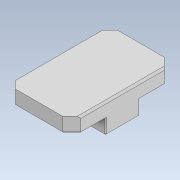
# Autodesk Inventor part: body_5
Saved by Autodesk Inventor 2020 (Build 240168000, 168)
## iProperties
Created: 2020-12-16
Part Number: body_5
Material: Generic
Document SubType Name: Modeling
Designer: DELL
Density: 1 g/cm^3
Appearance: Default
Mass: 2697.24 g
Surface Area: 1762.92 cm^2
Volume: 2697.24 cm^3
Author: DELL
Autodesk Inventor part; units mm, degrees
ref_plane "YZ Plane" through (0, 0, 0) normal (1, 0, 0) x (0, 1, 0)
ref_plane "XZ Plane" through (0, 0, 0) normal (0, 1, 0) x (-1, 0, 0)
ref_plane "XY Plane" through (0, 0, 0) normal (0, 0, 1) x (1, 0, 0)
sketch "Sketch1" plane through (0, 0, 0) normal (0, 1, 0) x (-1, 0, 0)
  line L0 (-90, -140) -> (90, -140)
  line L1 (90, -140) -> (90, 140)
  line L2 (90, 140) -> (-90, 140)
  line L3 (-90, 140) -> (-90, -140)
  line L4 (-90, -140) -> (90, 140) construction
  line L5 (90, -140) -> (-90, 140) construction
  point P0 (0, 0)
  dimension "d0" = 280
  dimension "d1" = 180
  constraints: 12 end point, 2 midpoint, 2 parallel, 1 horizontal, 1 perpendicular
  measures "d0" distance of L0.end L1.end
  measures "d1" distance between parallel lines of L3 L1
extrude "Extrusion1" add sketch "Sketch1" along normal blind 80
sketch "Sketch2" plane through (0, 0, 0) normal (0, -1, 0) x (1, 0, 0)
  arc A0 (-47.5, 47.5) -> (2.5, 97.5) centre (-47.5, 97.5) ccw
  line L0 (0, 150) -> (0, -153.5615) construction
  line L1 (-95.9498, 0) -> (75.0535, 0) construction
  line L2 (2.5, 97.5) -> (2.5, 140)
  line L3 (-90, 47.5) -> (-47.5, 47.5)
  line L4 (-90, -140) -> (-90, 140) projected
  line L5 (-90, 47.5) -> (-90, 140)
  line L6 (-90, 140) -> (90, 140) projected
  line L7 (2.5, 140) -> (-90, 140)
  arc A1 (-2.5, 97.5) -> (47.5, 47.5) centre (47.5, 97.5) ccw
  line L8 (-2.5, 97.5) -> (-2.5, 140)
  line L9 (90, 47.5) -> (47.5, 47.5)
  line L10 (90, -140) -> (90, 140)
  line L11 (90, 140) -> (-90, 140)
  arc A2 (2.5, -97.5) -> (-47.5, -47.5) centre (-47.5, -97.5) ccw
  line L12 (2.5, -97.5) -> (2.5, -140)
  line L13 (-90, -47.5) -> (-47.5, -47.5)
  line L14 (-90, 140) -> (-90, -140)
  line L15 (-90, -140) -> (90, -140)
  line L16 (90, 140) -> (90, -140)
  line L17 (90, -47.5) -> (47.5, -47.5)
  arc A3 (47.5, -47.5) -> (-2.5, -97.5) centre (47.5, -97.5) ccw
  line L18 (-2.5, -97.5) -> (-2.5, -140)
  circle A4 centre (-47.5, 97.5) radius 34.5
  circle A5 centre (-47.5, 97.5) radius 42 construction
  line L19 (-89.5, 97.5) -> (-5.5, 97.5) construction
  line L20 (-47.5, 139.5) -> (-47.5, 55.5) construction
  line L21 (-77.1985, 127.1985) -> (-17.8015, 67.8015) construction
  line L22 (-17.8015, 127.1985) -> (-77.1985, 67.8015) construction
  point P0 (0, 0)
  point P1 (-2.5, -140)
  point P2 (90, -47.5)
  point P3 (-90, -47.5)
  point P4 (-2.5, 140)
  point P5 (75, -50)
  point P6 (-75, -50)
  dimension "d15" = 84
  dimension "d7" = 90
  dimension "d11" = 50
  dimension "d14" = 69
  dimension "d16" = 45
  dimension "d17" = 45
  dimension "d35" = 42.5
  dimension "d36" = 42.5
  constraints: 42 end point, 23 symmetric about line, 8 point on circle, 7 midpoint, 6 point on line, 5 centre point, 4 vertical, 3 horizontal, 2 coincident, 2 tangent, 14 other
  measures "d7" angle of L3 L2
  measures "d11" radius of A0
  measures "d14" diameter of A4
  measures "d16" angle of L19 L21
  measures "d17" angle of L19 L22
  measures "d36" distance from line of L4 A0.centre
extrude "Extrusion2" cut sketch "Sketch2" against normal blind 40 contours L3 L4 L6 L8 A1 A0 | A1 L8 L6 L2 A0 | A0 L2 L6 L10 L9 A1 | L13 A2 A3 L18 L15 L4 | L10 L15 L12 A2 A3 L17 | L18 A3 A2 L12 L15 | A4
extrude "Extrusion3" cut sketch "Sketch2" against normal blind 12.5 from surface at -40 contours A4
mirror "Mirror1" about plane through (0, 0, 0) normal (0, 0, 1) of "Extrusion3"
mirror "Mirror2" about plane through (0, 0, 0) normal (1, 0, 0) of "Extrusion3", "Mirror1"
chamfer "Chamfer1" distance 25 angle 45 4 edges at (90, 60, 140) (-90, 60, 140) (90, 60, -140) (-90, 60, -140)
fillet "Fillet1" radius 20 2 edges at (0, 20, 81.8875) (0, 20, -81.8875)
chamfer "Chamfer2" distance 3 angle 45 26 edges at (0, 40, -140) (77.5, 40, -127.5) (90, 40, -81.25) (-77.5, 40, -127.5) (-90, 40, -81.25) (90, 40, 81.25) (77.5, 40, 127.5) (0, 40, 140) (-77.5, 40, 127.5) (-90, 40, 81.25) (-90, 0, 0) (-90, 20, 47.5) (-90, 20, -47.5) (-68.75, 0, -47.5) (-29.2837, 0, -50.9364) (0, 0, -66.0826) (29.2837, 0, -50.9364) (68.75, 0, -47.5) (-68.75, 0, 47.5) (-29.2837, 0, 50.9364) (0, 0, 66.0826) (29.2837, 0, 50.9364) (68.75, 0, 47.5) (90, 0, 0) (90, 20, -47.5) (90, 20, 47.5)
fillet "Fillet2" radius 3 8 edges at (29.2837, 40, -50.9364) (-29.2837, 40, -50.9364) (-67.25, 40, -47.5) (67.25, 40, -47.5) (29.2837, 40, 50.9364) (-29.2837, 40, 50.9364) (-67.25, 40, 47.5) (67.25, 40, 47.5)
chamfer "Chamfer4" distance 5 angle 45 2 edges at (90, 80, 0) (-90, 80, 0)
body "Solid1"
